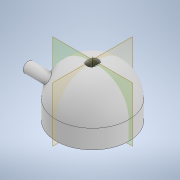
# Autodesk Inventor part: acoplamento joystick2
Saved by Autodesk Inventor 2022 (Build 260153000, 153)
## iProperties
Created: 2024-04-24
Part Number: acoplamento joystick2
Material: Generic
Document SubType Name: Modeling
Designer: admin
Density: 1 g/cm^3
Appearance: Default
Author: admin
Autodesk Inventor part; units mm, degrees
ref_plane "YZ Plane" through (0, 0, 0) normal (1, 0, 0) x (0, 1, 0)
ref_plane "XZ Plane" through (0, 0, 0) normal (0, 1, 0) x (-1, 0, 0)
ref_plane "XY Plane" through (0, 0, 0) normal (0, 0, 1) x (1, 0, 0)
sketch "Sketch1" plane through (0, 0, 0) normal (0, 1, 0) x (-1, 0, 0)
  circle A0 centre (0, 0) radius 14.5
  dimension "d0" = 29
  constraints: 1 centre point, 1 coincident
  measures "d0" diameter of A0
extrude "Extrusion1" add sketch "Sketch1" along normal blind 20
fillet "Fillet1" radius 12.5 1 edges at (14.5, 20, 0)
shell "Shell2" thickness 1 removed faces 0
sketch "Sketch6" plane through (0, 19, 0) normal (0, -1, 0) x (1, 0, 0)
  circle A0 centre (0, 0) radius 2 projected
  circle A1 centre (0, 0) radius 3
  dimension "d17" = 6
  constraints: 1 centre point, 1 coincident
  measures "d17" diameter of A1
extrude "Extrusion6" add sketch "Sketch6" along normal blind 6 contours A0 | A1
sketch "Sketch7" plane through (0, 20, 0) normal (0, 1, 0) x (1, 0, 0)
  circle A0 centre (0, 0) radius 2.3
  line L0 (-1.5775, 1.6738) -> (1.5775, 1.6738)
  line L1 (1.5775, 1.6738) -> (1.5775, -1.6738)
  line L2 (1.5775, -1.6738) -> (-1.5775, -1.6738)
  line L3 (-1.5775, -1.6738) -> (-1.5775, 1.6738)
  line L4 (-1.5775, 1.6738) -> (1.5775, -1.6738) construction
  line L5 (1.5775, 1.6738) -> (-1.5775, -1.6738) construction
  dimension "d20" = 4.6
  constraints: 12 end point, 2 midpoint, 2 parallel, 1 coincident, 1 horizontal, 1 perpendicular, 3 other
extrude "Extrusion7" cut sketch "Sketch7" against normal blind 5 contours L0 A0 | L1 L2 L3 L0 | A0 L2
sketch "Sketch12" plane through (0, 0, 0) normal (0, -1, 0) x (1, 0, 0)
  circle A0 centre (0, 0) radius 13.5
  dimension "d48" = 27
  constraints: 1 centre point, 1 coincident
  measures "d48" diameter of A0
extrude "Extrusion12" add sketch "Sketch12" against normal blind 12
ref_plane "Work Plane1" through (0, 20, 0) normal (0, 0, -1) x (0, -1, 0)
sketch "Sketch14" plane through (0, 20, 0) normal (0, 0, -1) x (0, -1, 0)
  line L0 (20, 0) -> (18, 0)
  line L1 (18, 0) -> (18, 3.2)
  line L2 (18, 3.2) -> (20, 3.2)
  line L3 (20, 3.2) -> (20, 0)
  line L4 (18, 0) -> (18, 2.5)
  line L5 (18, 0) -> (8, 0)
  line L6 (8, 0) -> (8, 2.15)
  line L7 (18, 2.5) -> (8, 2.15)
  line L8 (-4.0048, 0) -> (24.0008, 0) projected
  dimension "d55" = 2
  dimension "d56" = 3.2
  dimension "d57" = 2.5
  dimension "d58" = 10
  dimension "d59" = 2.15
  constraints: 16 end point, 3 perpendicular, 2 parallel, 1 horizontal, 1 point on line
  measures "d55" distance of L1.end L2.end
  measures "d56" distance of L0.end L1.end
  measures "d57" distance of L0.end L4.end
  measures "d58" distance of L0.end L5.end
  measures "d59" distance of L5.end L6.end
revolve "Revolution1" cut sketch "Sketch14" angle 360 about axis through (0, 20, 0) along (0, 1, 0)
ref_plane "Work Plane2" through (0, 20, 0) normal (1, 0, 0) x (0, -1, 0)
sketch "Sketch16" plane through (0, 20, 0) normal (1, 0, 0) x (0, -1, 0)
  line L0 (20, 0) -> (6.7037, 0)
  line L1 (6.7037, 0) -> (6.7037, -7.6663)
  line L2 (6.7037, -7.6663) -> (20, -7.6663)
  line L3 (20, -7.6663) -> (20, 0)
  circle A0 centre (6.7037, -7.6663) radius 2.1
  circle A1 centre (6.7037, -7.6663) radius 1
  dimension "d62" = 4.2
  dimension "d63" = 2
  constraints: 8 end point, 2 centre point, 2 coincident, 2 parallel, 1 horizontal, 1 perpendicular
  measures "d62" diameter of A0
  measures "d63" diameter of A1
extrude "Extrusion14" cut sketch "Sketch16" against normal blind 15 contours A1 L2 L1 | L1 L2 A1
extrude "Extrusion15" add sketch "Sketch16" against normal blind 18 contours A0 L2 A1 L1 | L1 A1 L2 A0
body "Solid1"
